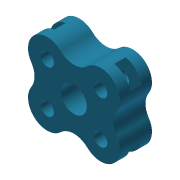
# Autodesk Inventor part: PlateAttache
Saved by Autodesk Inventor 2014 (Build 180170000, 170)
## iProperties
Created: 2014-09-17
Part Number: PlateAttache
Material: Generic
Document SubType Name: Modeling
Designer: Peele
Density: 1 g/cm^3
Appearance: Turquoise
Author: Peele
Autodesk Inventor part; units mm, degrees
ref_plane "YZ Plane" through (0, 0, 0) normal (1, 0, 0) x (0, 1, 0)
ref_plane "XZ Plane" through (0, 0, 0) normal (0, 1, 0) x (-1, 0, 0)
ref_plane "XY Plane" through (0, 0, 0) normal (0, 0, 1) x (1, 0, 0)
sketch "Sketch1" plane through (0, 0, 0) normal (0, 1, 0) x (-1, 0, 0)
  line L0 (-12.5, -10) -> (12.5, -10) construction
  line L1 (12.5, -10) -> (12.5, 10) construction
  line L2 (12.5, 10) -> (-12.5, 10) construction
  line L3 (-12.5, 10) -> (-12.5, -10) construction
  line L4 (-12.5, -10) -> (12.5, 10) construction
  line L5 (12.5, -10) -> (-12.5, 10) construction
  circle A0 centre (-12.5, 10) radius 3.1
  circle A1 centre (12.5, 10) radius 3.1
  circle A2 centre (12.5, -10) radius 3.1
  circle A3 centre (-12.5, -10) radius 3.1
  circle A4 centre (-12.5, 10) radius 6.5 construction
  circle A5 centre (12.5, 10) radius 6.5 construction
  circle A6 centre (-12.5, -10) radius 6.5 construction
  circle A7 centre (0, 0) radius 6
  arc A8 (-6.25, 16.4759) -> (-19.9833, 5) centre (-12.5, 10) ccw
  arc A9 (-6.25, 16.4759) -> (6.25, 16.4759) centre (0, 22.9518) ccw
  arc A10 (19.9833, 5) -> (6.25, 16.4759) centre (12.5, 10) ccw
  arc A11 (19.9833, 5) -> (19.9833, -5) centre (27.4666, 0) ccw
  arc A12 (6.25, -16.4759) -> (19.9833, -5) centre (12.5, -10) ccw
  arc A13 (6.25, -16.4759) -> (-6.25, -16.4759) centre (0, -22.9518) ccw
  arc A14 (-19.9833, -5) -> (-6.25, -16.4759) centre (-12.5, -10) ccw
  arc A15 (-19.9833, -5) -> (-19.9833, 5) centre (-27.4666, 0) ccw
  dimension "d0" = 6.2
  dimension "d1" = 13
  dimension "d2" = 20
  dimension "d4" = 12
  dimension "d5" = 25
  dimension "d9" = 9
  dimension "d10" = 9
  dimension "d11" = 9
  constraints: 18 equal radius, 16 centre point, 16 point on circle, 12 end point, 8 coincident, 4 concentric, 2 horizontal alignment, 2 midpoint, 2 parallel, 1 horizontal, 1 perpendicular
  measures "d0" diameter of A0
  measures "d1" diameter of A4
  measures "d2" distance of L2.end L0.start
  measures "d4" diameter of A7
  measures "d5" distance of L1.end L2.end
  measures "d9" radius of A8
  measures "d10" radius of A11
  measures "d11" radius of A13
extrude "Extrusion1" add sketch "Sketch1" along normal mid plane 15
sketch "Sketch2" plane through (0, 0, 0) normal (0, 1, 0) x (-1, 0, 0)
  line L0 (-16.7866, 14.2866) -> (-10.931, 15.8556) construction
  line L1 (-10.931, 15.8556) -> (-6.6444, 11.569)
  line L2 (-6.6444, 11.569) -> (-8.2134, 5.7134)
  line L3 (-8.2134, 5.7134) -> (-14.069, 4.1444)
  line L4 (-14.069, 4.1444) -> (-18.3556, 8.431)
  line L5 (-18.3556, 8.431) -> (-16.7866, 14.2866) construction
  line L6 (-18.3556, 8.431) -> (-28.3556, 18.431)
  line L7 (-28.3556, 18.431) -> (-20.931, 25.8556)
  line L8 (-20.931, 25.8556) -> (-10.931, 15.8556)
  circle A0 centre (-12.5, 10) radius 3.1 projected
  circle A1 centre (12.5, 10) radius 3.1 projected
  circle A2 centre (12.5, -10) radius 3.1 projected
  circle A3 centre (-12.5, -10) radius 3.1 projected
  line L9 (0, 0) -> (-12.5, 10) construction
  line L10 (0, 0) -> (-26.3012, 0) construction
  line L11 (16.7866, 14.2866) -> (18.3556, 8.431) construction
  line L12 (18.3556, 8.431) -> (14.069, 4.1444)
  line L13 (14.069, 4.1444) -> (8.2134, 5.7134)
  line L14 (8.2134, 5.7134) -> (6.6444, 11.569)
  line L15 (6.6444, 11.569) -> (10.931, 15.8556)
  line L16 (10.931, 15.8556) -> (16.7866, 14.2866) construction
  line L17 (16.7866, -14.2866) -> (10.931, -15.8556) construction
  line L18 (10.931, -15.8556) -> (6.6444, -11.569)
  line L19 (6.6444, -11.569) -> (8.2134, -5.7134)
  line L20 (8.2134, -5.7134) -> (14.069, -4.1444)
  line L21 (14.069, -4.1444) -> (18.3556, -8.431)
  line L22 (18.3556, -8.431) -> (16.7866, -14.2866) construction
  line L23 (-16.7866, -14.2866) -> (-18.3556, -8.431) construction
  line L24 (-18.3556, -8.431) -> (-14.069, -4.1444)
  line L25 (-14.069, -4.1444) -> (-8.2134, -5.7134)
  line L26 (-8.2134, -5.7134) -> (-6.6444, -11.569)
  line L27 (-6.6444, -11.569) -> (-10.931, -15.8556)
  line L28 (-10.931, -15.8556) -> (-16.7866, -14.2866) construction
  line L29 (10.931, 15.8556) -> (20.931, 25.8556)
  line L30 (20.931, 25.8556) -> (28.3556, 18.431)
  line L31 (28.3556, 18.431) -> (18.3556, 8.431)
  line L32 (18.3556, -8.431) -> (28.3556, -18.431)
  line L33 (28.3556, -18.431) -> (20.931, -25.8556)
  line L34 (20.931, -25.8556) -> (10.931, -15.8556)
  line L35 (-10.931, -15.8556) -> (-20.931, -25.8556)
  line L36 (-20.931, -25.8556) -> (-28.3556, -18.431)
  line L37 (-28.3556, -18.431) -> (-18.3556, -8.431)
  dimension "d12" = 10.5
  dimension "d13" = 45
  dimension "d14" = 45
  dimension "d15" = 10
  constraints: 76 end point, 6 equal length, 6 perpendicular, 4 coincident, 3 collinear, 3 parallel, 2 horizontal alignment, 1 horizontal, 52 other
  measures "d12" distance between parallel lines of L4 L1
  measures "d13" angle of L6 L10
  measures "d14" angle of L10 L24
  measures "d15" horizontal distance of L7.end L0.end
extrude "Extrusion2" cut sketch "Sketch2" along normal mid plane 5.25
body "Solid1"
